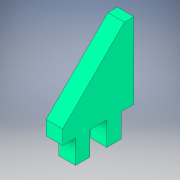
# Autodesk Inventor part: MonsterHolderSupport1
Saved by Autodesk Inventor 2019 (Build 230136000, 136)
## iProperties
Created: 2018-12-04
Part Number: MonsterHolderSupport1
Material: Generic
Document SubType Name: Modeling
Designer: Administrator
Density: 1 g/cm^3
Appearance: Default
Author: Administrator
Autodesk Inventor part; units mm, degrees
ref_plane "YZ Plane" through (0, 0, 0) normal (1, 0, 0) x (0, 1, 0)
ref_plane "XZ Plane" through (0, 0, 0) normal (0, 1, 0) x (-1, 0, 0)
ref_plane "XY Plane" through (0, 0, 0) normal (0, 0, 1) x (1, 0, 0)
sketch "Sketch1" plane through (0, 0, 0) normal (0, 0, 1) x (1, 0, 0)
  line L0 (0, 0) -> (4.445, 0)
  line L1 (4.445, 0) -> (4.445, 20.32)
  line L2 (4.445, 20.32) -> (0, 20.32)
  line L3 (0, 20.32) -> (0, 0)
  dimension "d0" = 4.445
  dimension "d1" = 20.32
  constraints: 8 end point, 2 parallel, 1 horizontal, 1 perpendicular
  measures "d0" distance of L1.end L2.end
  measures "d1" distance of L0.end L1.end
extrude "Extrusion1" add sketch "Sketch1" along normal blind 19.05
chamfer "Chamfer1" distance 16.51 angle 45 1 edges at (2.2225, 20.32, 19.05)
sketch "Sketch2" plane through (0, 0, 0) normal (0, -1, 0) x (1, 0, 0)
  line L0 (0, 19.05) -> (4.445, 19.05) projected
  line L1 (0, 0) -> (4.445, 0) projected
  line L2 (0, 3.429) -> (4.445, 3.429)
  line L3 (4.445, 3.429) -> (4.445, 7.239)
  line L4 (4.445, 7.239) -> (0, 7.239)
  line L5 (0, 7.239) -> (0, 3.429)
  line L6 (4.445, 0) -> (4.445, 19.05) projected
  line L7 (0, 11.811) -> (4.445, 11.811)
  line L8 (4.445, 11.811) -> (4.445, 15.621)
  line L9 (4.445, 15.621) -> (0, 15.621)
  line L10 (0, 15.621) -> (0, 11.811)
  dimension "d7" = 19.05
  dimension "d8" = 3.81
  dimension "d9" = 3.81
  dimension "d10" = 4.445
  dimension "d11" = 4.445
  dimension "d12" = 3.429
  dimension "d13" = 3.429
  dimension "d16" = 8.382
  constraints: 16 end point, 4 parallel, 2 horizontal, 2 perpendicular, 2 point on line
  measures "d7" distance between parallel lines of L0 L1
  measures "d8" distance of L9.end L7.start
  measures "d9" distance of L4.end L2.start
  measures "d10" distance of L2.start L2.end
  measures "d11" distance of L7.start L7.end
  measures "d12" distance between parallel lines of L0 L9
  measures "d13" distance between parallel lines of L1 L2
  measures "d16" distance between parallel lines of L4 L9
extrude "Extrusion2" add sketch "Sketch2" along normal blind 6.35
body "Solid1"
